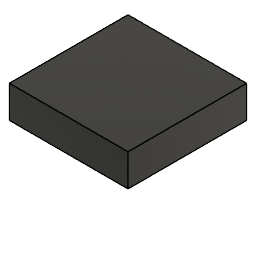
piston (Autodesk Fusion 360 design; units mm, degrees)
part number: 2026-06-04-20-41-35-303
Autodesk Fusion 360 part; units mm, degrees
sketch "Sketch1" plane through (0, 0, 0) normal (0, 0, 1) x (1, 0, 0)
  line L0 (0, 0) -> (0, 77.5)
  line L1 (0, 77.5) -> (55.5, 77.5)
  line L2 (55.5, 77.5) -> (55.5, -0.5)
  line L3 (55.5, -0.5) -> (133, -0.5)
  line L4 (133, -0.5) -> (133, -56)
  line L5 (133, -56) -> (55.5, -56)
  line L6 (55.5, -56) -> (55.5, -133.5)
  line L7 (55.5, -133.5) -> (0, -133.5)
  line L8 (0, -133.5) -> (0, -56)
  line L9 (0, -56) -> (-77.5, -56)
  line L10 (-77.5, -56) -> (-77.5, 0)
  line L11 (-77.5, 0) -> (0, 0)
  dimension "d1" = 77.5
  dimension "d2" = 55.5
  dimension "d3" = 77.5
  dimension "d4" = 55.5
  dimension "d5" = 77.5
  dimension "d6" = 77.5
  dimension "d7" = 55.5
  dimension "d8" = 77.5
  dimension "d9" = 77.5
  constraint coincident L0.start L11.end
  constraint vertical L0
  constraint perpendicular L0 L1
  constraint perpendicular L1 L2
  constraint perpendicular L2 L3
  constraint perpendicular L3 L4
  constraint perpendicular L4 L5
  constraint perpendicular L5 L6
  constraint perpendicular L6 L7
  constraint perpendicular L7 L8
  constraint perpendicular L8 L9
  constraint perpendicular L9 L10
  constraint perpendicular L0 L11
  measures "d1" distance of L0.start L0.end
  measures "d2" distance of L0.end L1.end
  measures "d3" distance of L2.end L3.end
  measures "d4" distance of L3.end L4.end
  measures "d5" distance of L4.end L5.end
  measures "d6" distance of L5.end L6.end
  measures "d7" distance of L6.end L7.end
  measures "d8" distance of L7.end L8.end
  measures "d9" distance of L8.end L9.end
extrude "Extrude1" add sketch "Sketch1" along normal blind 250
sketch "Sketch2" plane through (0, 0, 250) normal (0, 0, 1) x (-1, 0, 0)
  line L0 (77.5, 0) -> (77.5, 56)
  line L1 (77.5, 56) -> (0, 56)
  line L2 (0, 56) -> (0, 133.5)
  line L3 (0, 133.5) -> (-55.5, 133.5)
  line L4 (-55.5, 133.5) -> (-55.5, 56)
  line L5 (-55.5, 56) -> (-133, 56)
  line L6 (-133, 56) -> (-133, 0.5)
  line L7 (-133, 0.5) -> (-55.5, 0.5)
  line L8 (-55.5, 0.5) -> (-55.5, -77.5)
  line L9 (-55.5, -77.5) -> (0, -77.5)
  line L10 (0, -77.5) -> (0, 0)
  line L11 (0, 0) -> (77.5, 0)
  line L12 (267.25, -267) -> (-322.75, -267)
  line L13 (-322.75, -267) -> (-322.75, 323)
  line L14 (-322.75, 323) -> (267.25, 323)
  line L15 (267.25, 323) -> (267.25, -267)
  line L16 (267.25, -267) -> (-322.75, 323) construction
  line L17 (-322.75, -267) -> (267.25, 323) construction
  line L18 (0, 0) -> (-55.5, 0) construction
  line L19 (-55.5, 0) -> (-55.5, 56) construction
  line L20 (-55.5, 56) -> (0, 56) construction
  line L21 (0, 56) -> (0, 0) construction
  line L22 (0, 0) -> (-55.5, 56) construction
  line L23 (-55.5, 0) -> (0, 56) construction
  point P0 (-27.75, 28)
  point P1 (-27.75, 28)
  dimension "d12" = 590
  dimension "d13" = 590
  constraint horizontal L12
  constraint vertical L13
  constraint horizontal L14
  constraint vertical L15
  constraint midpoint L17 P1
  constraint horizontal L18
  constraint vertical L19
  constraint horizontal L20
  constraint vertical L21
  constraint coincident L4.end L5.start
  constraint coincident L10.end L11.start
  constraint midpoint L23 P1
  constraint coincident P1 P0
  measures "d12" distance of L12.start L14.end
  measures "d13" distance of L12.start L12.end
extrude "Extrude2" add sketch "Sketch2" along normal blind 160 contours L0 L1 L2 L3 L4 L5 L6 L7 L8 L9 L10 L11 | L12 L13 L14 L15
ref_plane "WorkPlane1" through (0, -25, 0) normal (0, 1, 0) x (0, 0, 1)
sketch "Sketch3" plane through (0, -25, 0) normal (0, 1, 0) x (1, 0, 0)
  spline S0 degree 5 poles (-27.9354, -72.4403) (-25.9191, -69.4136) (-21.8921, -63.6238) (-15.8685, -55.7292) (-7.8716, -46.8098) (2.0631, -38.5208) (11.9309, -33.3508) (21.7262, -31.5591) (31.4458, -33.2959) (41.0924, -38.4323) (50.6714, -46.7164) (58.285, -55.6575) (63.969, -63.5825) (67.7468, -69.3988) (69.6329, -72.4403) knots 0 0 0 0 0 0 0.1 0.2 0.3 0.4 0.5 0.6 0.7 0.8 0.9 1 1 1 1 1 1
  point P0 (22.0646, -32.4403)
pipe "Pipe1" add diameter 10 path "Sketch3" along S0
extrude "Extrude3" cut sketch "Sketch1" along normal blind 75
pipe "Pipe2" add diameter 15 path "Sketch3" along S0
scale "Scale1" factor 0.254237 about (322.75, 267, 410) bodies 1
extrude "Extrude4" add 1 faces at (233.7711, 192.2043, 324.2986) along direction (-0.554428, 0, 0.832232) blind 2
extrude "Extrude5" add 1 faces at (259.3259, 192.757, 323.6045) along direction (0.52702, 0, 0.849853) blind 5
